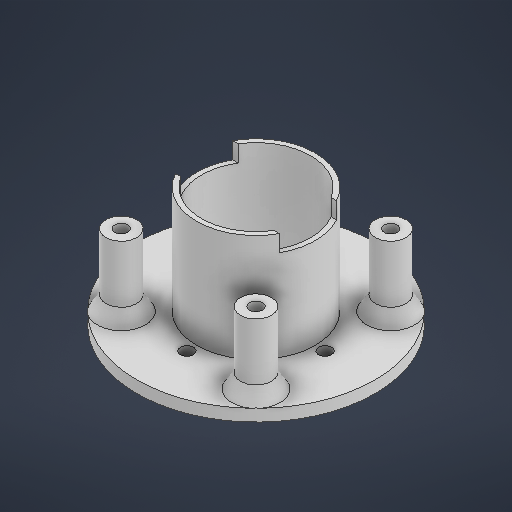
# Autodesk Inventor part: holder
Saved by Autodesk Inventor 2025 (Build 290162000, 162)
## iProperties
Created: 2024-10-04
Part Number: holder
Material: Generic
Document SubType Name: Modeling
Designer: mayhe
Density: 1 g/cm^3
Appearance: Default
Author: mayhe
Autodesk Inventor part; units mm, degrees
ref_plane "YZ Plane" through (0, 0, 0) normal (1, 0, 0) x (0, 1, 0)
ref_plane "XZ Plane" through (0, 0, 0) normal (0, 1, 0) x (-1, 0, 0)
ref_plane "XY Plane" through (0, 0, 0) normal (0, 0, 1) x (1, 0, 0)
sketch "Sketch1" plane through (0, 0, 0) normal (0, 1, 0) x (-1, 0, 0)
  circle A0 centre (0, 0) radius 50
  circle A1 centre (0, 0) radius 40
  circle A2 centre (0, -40) radius 2.75
  circle A3 centre (28.2843, -28.2843) radius 2.75
  circle A4 centre (40, 0) radius 2.75
  circle A5 centre (28.2843, 28.2843) radius 2.75
  circle A6 centre (0, 0) radius 22.9
  circle A7 centre (0, 0) radius 24.9
  line L0 (31.0901, 12) -> (-31.0901, 12)
  line L1 (-31.0901, 12) -> (-31.0901, -12)
  line L2 (-31.0901, -12) -> (31.0901, -12)
  line L3 (31.0901, -12) -> (31.0901, 12)
  line L4 (31.0901, 12) -> (-31.0901, -12) construction
  line L5 (-31.0901, 12) -> (31.0901, -12) construction
  circle A8 centre (0, 40) radius 2.75
  circle A9 centre (-28.2843, 28.2843) radius 2.75
  circle A10 centre (-40, 0) radius 2.75
  circle A11 centre (-28.2843, -28.2843) radius 2.75
  point P0 (-21.8177, 12)
  point P1 (-19.5041, 12)
  point P2 (19.5041, 12)
  point P3 (21.8177, 12)
  point P4 (21.8177, -12)
  point P5 (19.5041, -12)
  point P6 (-19.5041, -12)
  point P7 (-21.8177, -12)
  dimension "d1" = 80
  dimension "d0" = 100
  dimension "d2" = 5.5
  dimension "d5" = 360
  dimension "d7" = 45.8
  dimension "d8" = 2
  dimension "d9" = 24
  constraints: 12 end point, 11 centre point, 3 coincident, 2 midpoint, 2 parallel, 1 horizontal, 1 perpendicular, 1 vertical alignment, 19 other
  measures "d0" diameter of A0
  measures "d2" diameter of A2
  measures "d7" diameter of A6
  measures "d8" radial gap between concentric circles of A6 A7
  measures "d9" distance of L1.end L0.end
extrude "Extrusion1" add sketch "Sketch1" along normal blind 5 contours A0 | A1 A4 | A1 A4 | A4 A1 A3 A2 A11 A10 A9 A8 A5 | A8 A1 | A1 A8 | A2 A1 | A1 A2 | A10 A1 | A1 A10 | A6 L2 L0 | A6 L0 A7 L2 | L0 A6 | A6 L0 A7 | L2 A7 A6 | A6 L2 | A6 L2 A7 L0 | L0 L3 L2 A7 | A7 L2 L1 L0
extrude "Extrusion2" add sketch "Sketch1" along normal blind 50.1 contours A6 L0 A7 | L2 A7 A6
extrude "Extrusion3" add sketch "Sketch1" along normal blind 43.1 contours A6 L0 A7 L2 | A6 L2 A7 L0
sketch "Sketch2" plane through (0, 5, 0) normal (0, 1, 0) x (1, 0, 0)
  circle A0 centre (0, 0) radius 29
  circle A1 centre (29, 0) radius 2.75
  circle A2 centre (0, 29) radius 2.75
  circle A3 centre (-29, 0) radius 2.75
  circle A4 centre (0, -29) radius 2.75
  dimension "d16" = 58
  dimension "d17" = 5.5
  dimension "d20" = 360
  constraints: 4 centre point, 1 coincident, 1 horizontal alignment, 11 other
  measures "d17" diameter of A1
extrude "Extrusion4" cut sketch "Sketch2" against normal blind 43.1 contours A0 A1 | A0 A1 | A2 A0 | A0 A2 | A4 A0 | A0 A4 | A3 A0 | A0 A3
sketch "Sketch3" plane through (0, 5, 0) normal (0, 1, 0) x (1, 0, 0)
  circle A0 centre (-28.2843, 28.2843) radius 2.75 projected
  circle A1 centre (0, 0) radius 40
  circle A2 centre (0, 40) radius 6.5
  circle A3 centre (0, 40) radius 4
  line L0 (2.3094, 44) -> (4.6188, 40)
  line L1 (4.6188, 40) -> (2.3094, 36)
  line L2 (2.3094, 36) -> (-2.3094, 36)
  line L3 (-2.3094, 36) -> (-4.6188, 40)
  line L4 (-4.6188, 40) -> (-2.3094, 44)
  line L5 (-2.3094, 44) -> (2.3094, 44)
  circle A4 centre (-28.2843, 28.2843) radius 6.5
  line L6 (-29.4797, 32.7457) -> (-25.0183, 31.5503)
  line L7 (-32.7457, 29.4797) -> (-29.4797, 32.7457)
  line L8 (-31.5503, 25.0183) -> (-32.7457, 29.4797)
  circle A5 centre (-28.2843, 28.2843) radius 4
  line L9 (-25.0183, 31.5503) -> (-23.8229, 27.0888)
  line L10 (-23.8229, 27.0888) -> (-27.0888, 23.8229)
  line L11 (-27.0888, 23.8229) -> (-31.5503, 25.0183)
  circle A6 centre (-40, 0) radius 6.5
  line L12 (-44, 2.3094) -> (-40, 4.6188)
  line L13 (-44, -2.3094) -> (-44, 2.3094)
  line L14 (-40, -4.6188) -> (-44, -2.3094)
  circle A7 centre (-40, 0) radius 4
  line L15 (-40, 4.6188) -> (-36, 2.3094)
  line L16 (-36, 2.3094) -> (-36, -2.3094)
  line L17 (-36, -2.3094) -> (-40, -4.6188)
  circle A8 centre (-28.2843, -28.2843) radius 6.5
  line L18 (-32.7457, -29.4797) -> (-31.5503, -25.0183)
  line L19 (-29.4797, -32.7457) -> (-32.7457, -29.4797)
  line L20 (-25.0183, -31.5503) -> (-29.4797, -32.7457)
  circle A9 centre (-28.2843, -28.2843) radius 4
  line L21 (-31.5503, -25.0183) -> (-27.0888, -23.8229)
  line L22 (-27.0888, -23.8229) -> (-23.8229, -27.0888)
  line L23 (-23.8229, -27.0888) -> (-25.0183, -31.5503)
  circle A10 centre (0, -40) radius 6.5
  line L24 (-2.3094, -44) -> (-4.6188, -40)
  line L25 (2.3094, -44) -> (-2.3094, -44)
  line L26 (4.6188, -40) -> (2.3094, -44)
  circle A11 centre (0, -40) radius 4
  line L27 (-4.6188, -40) -> (-2.3094, -36)
  line L28 (-2.3094, -36) -> (2.3094, -36)
  line L29 (2.3094, -36) -> (4.6188, -40)
  circle A12 centre (28.2843, -28.2843) radius 6.5
  line L30 (29.4797, -32.7457) -> (25.0183, -31.5503)
  line L31 (32.7457, -29.4797) -> (29.4797, -32.7457)
  line L32 (31.5503, -25.0183) -> (32.7457, -29.4797)
  circle A13 centre (28.2843, -28.2843) radius 4
  line L33 (25.0183, -31.5503) -> (23.8229, -27.0888)
  line L34 (23.8229, -27.0888) -> (27.0888, -23.8229)
  line L35 (27.0888, -23.8229) -> (31.5503, -25.0183)
  circle A14 centre (40, 0) radius 6.5
  line L36 (44, -2.3094) -> (40, -4.6188)
  line L37 (44, 2.3094) -> (44, -2.3094)
  line L38 (40, 4.6188) -> (44, 2.3094)
  circle A15 centre (40, 0) radius 4
  line L39 (40, -4.6188) -> (36, -2.3094)
  line L40 (36, -2.3094) -> (36, 2.3094)
  line L41 (36, 2.3094) -> (40, 4.6188)
  circle A16 centre (28.2843, 28.2843) radius 6.5
  line L42 (32.7457, 29.4797) -> (31.5503, 25.0183)
  line L43 (29.4797, 32.7457) -> (32.7457, 29.4797)
  line L44 (25.0183, 31.5503) -> (29.4797, 32.7457)
  circle A17 centre (28.2843, 28.2843) radius 4
  line L45 (31.5503, 25.0183) -> (27.0888, 23.8229)
  line L46 (27.0888, 23.8229) -> (23.8229, 27.0888)
  line L47 (23.8229, 27.0888) -> (25.0183, 31.5503)
  circle A18 centre (40, 0) radius 2.75
  circle A19 centre (28.2843, 28.2843) radius 2.75
  circle A20 centre (0, 40) radius 2.75
  circle A21 centre (-28.2843, 28.2843) radius 2.75
  circle A22 centre (-40, 0) radius 2.75
  circle A23 centre (-28.2843, -28.2843) radius 2.75
  circle A24 centre (0, -40) radius 2.75
  circle A25 centre (28.2843, -28.2843) radius 2.75
  point P0 (0, 44)
  point P1 (-31.1127, 31.1127)
  point P2 (-44, 0)
  point P3 (-31.1127, -31.1127)
  point P4 (0, -44)
  point P5 (31.1127, -31.1127)
  point P6 (44, 0)
  point P7 (31.1127, 31.1127)
  point P8 (-4.4739, 39.749)
  point P9 (-3.4641, 38)
  point P10 (-3.995, 39.8)
  dimension "d29" = 8
  dimension "d24" = 13
  dimension "d36" = 360
  dimension "d38" = 5.5
  dimension "d41" = 360
  constraints: 96 end point, 17 centre point, 11 coincident, 2 horizontal alignment, 2 point on circle, 1 midpoint, 1 vertical alignment, 188 other
  measures "d24" diameter of A2
  measures "d38" diameter of A18
extrude "Extrusion5" add sketch "Sketch3" along normal blind 15 contours A0 A1 A5 | A0 A1 A5 | A5 L6 L9 A1 | A1 L9 A5 | A5 L11 A1 | A1 L11 L8 A5 | L9 L6 L7 L8 L11 A1 A4 | A1 A4 L11 L10 L9 | L9 L10 A5 | A5 L7 L6 | L8 L7 A5 | A5 L10 L11 | A16 A1 L45 L42 L43 L44 L47 | A1 L47 L46 L45 A16 | A8 A1 L23 L22 L21 | A1 L21 L18 L19 L20 L23 A8 | L47 L44 A17 A1 | A1 A17 L47 | L21 A9 A1 | A1 A9 L18 L21 | A17 A1 A19 | A1 A19 A17 | A17 L46 L47 | L45 A17 A1 | A1 A17 L42 L45 | A9 A1 A23 | A1 A23 A9 | L21 L22 A9 | L23 L20 A9 A1 | A1 A9 L23 | L44 L43 A17 | A17 L45 L46 | A9 L19 L18 | L22 L23 A9 | L43 L42 A17 | A12 A1 L33 L30 L31 L32 L35 | A1 L35 L34 L33 A12 | A9 L20 L19 | L35 L32 A13 A1 | A1 A13 L35 | L33 A13 A1 | A1 A13 L30 L33 | A13 A1 A25 | A1 A25 A13 | A13 L34 L35 | L33 L34 A13 | L32 L31 A13 | A13 L31 L30
sketch "Sketch4" plane through (28.2843, 20, 28.2843) normal (0, 1, 0) x (1, 0, 0)
  circle A0 centre (0, 0) radius 6.5 projected
  circle A1 centre (0, 0) radius 6.5
  circle A2 centre (0, 0) radius 4
  circle A3 centre (0, 0) radius 2.75
  line L0 (4, -2.3094) -> (0, -4.6188)
  line L1 (0, -4.6188) -> (-4, -2.3094)
  line L2 (-4, -2.3094) -> (-4, 2.3094)
  line L3 (-4, 2.3094) -> (0, 4.6188)
  line L4 (0, 4.6188) -> (4, 2.3094)
  line L5 (4, 2.3094) -> (4, -2.3094)
  circle A4 centre (-28.2843, 28.2843) radius 40
  circle A5 centre (11.7157, 28.2843) radius 6.5
  line L6 (8.4497, 31.5503) -> (12.9112, 32.7457)
  line L7 (7.2543, 27.0888) -> (8.4497, 31.5503)
  line L8 (10.5203, 23.8229) -> (7.2543, 27.0888)
  line L9 (14.9817, 25.0183) -> (10.5203, 23.8229)
  line L10 (16.1771, 29.4797) -> (14.9817, 25.0183)
  line L11 (12.9112, 32.7457) -> (16.1771, 29.4797)
  circle A6 centre (11.7157, 28.2843) radius 2.75
  circle A7 centre (0, 56.5685) radius 6.5
  line L12 (-4.6188, 56.5685) -> (-2.3094, 60.5685)
  line L13 (-2.3094, 52.5685) -> (-4.6188, 56.5685)
  line L14 (2.3094, 52.5685) -> (-2.3094, 52.5685)
  line L15 (4.6188, 56.5685) -> (2.3094, 52.5685)
  line L16 (2.3094, 60.5685) -> (4.6188, 56.5685)
  line L17 (-2.3094, 60.5685) -> (2.3094, 60.5685)
  circle A8 centre (0, 56.5685) radius 2.75
  circle A9 centre (-28.2843, 68.2843) radius 6.5
  line L18 (-31.5503, 65.0183) -> (-32.7457, 69.4797)
  line L19 (-27.0888, 63.8229) -> (-31.5503, 65.0183)
  line L20 (-23.8229, 67.0888) -> (-27.0888, 63.8229)
  line L21 (-25.0183, 71.5503) -> (-23.8229, 67.0888)
  line L22 (-29.4797, 72.7457) -> (-25.0183, 71.5503)
  line L23 (-32.7457, 69.4797) -> (-29.4797, 72.7457)
  circle A10 centre (-28.2843, 68.2843) radius 2.75
  circle A11 centre (-56.5685, 56.5685) radius 6.5
  line L24 (-56.5685, 51.9497) -> (-60.5685, 54.2591)
  line L25 (-52.5685, 54.2591) -> (-56.5685, 51.9497)
  line L26 (-52.5685, 58.8779) -> (-52.5685, 54.2591)
  line L27 (-56.5685, 61.1873) -> (-52.5685, 58.8779)
  line L28 (-60.5685, 58.8779) -> (-56.5685, 61.1873)
  line L29 (-60.5685, 54.2591) -> (-60.5685, 58.8779)
  circle A12 centre (-56.5685, 56.5685) radius 2.75
  circle A13 centre (-68.2843, 28.2843) radius 6.5
  line L30 (-65.0183, 25.0183) -> (-69.4797, 23.8229)
  line L31 (-63.8229, 29.4797) -> (-65.0183, 25.0183)
  line L32 (-67.0888, 32.7457) -> (-63.8229, 29.4797)
  line L33 (-71.5503, 31.5503) -> (-67.0888, 32.7457)
  line L34 (-72.7457, 27.0888) -> (-71.5503, 31.5503)
  line L35 (-69.4797, 23.8229) -> (-72.7457, 27.0888)
  circle A14 centre (-68.2843, 28.2843) radius 2.75
  circle A15 centre (-56.5685, 0) radius 6.5
  line L36 (-51.9497, 0) -> (-54.2591, -4)
  line L37 (-54.2591, 4) -> (-51.9497, 0)
  line L38 (-58.8779, 4) -> (-54.2591, 4)
  line L39 (-61.1873, 0) -> (-58.8779, 4)
  line L40 (-58.8779, -4) -> (-61.1873, 0)
  line L41 (-54.2591, -4) -> (-58.8779, -4)
  circle A16 centre (-56.5685, 0) radius 2.75
  circle A17 centre (-28.2843, -11.7157) radius 6.5
  line L42 (-25.0183, -8.4497) -> (-23.8229, -12.9112)
  line L43 (-29.4797, -7.2543) -> (-25.0183, -8.4497)
  line L44 (-32.7457, -10.5203) -> (-29.4797, -7.2543)
  line L45 (-31.5503, -14.9817) -> (-32.7457, -10.5203)
  line L46 (-27.0888, -16.1771) -> (-31.5503, -14.9817)
  line L47 (-23.8229, -12.9112) -> (-27.0888, -16.1771)
  circle A18 centre (-28.2843, -11.7157) radius 2.75
  point P0 (4, 0)
  point P1 (14.5442, 31.1127)
  point P2 (0, 60.5685)
  point P3 (-31.1127, 71.1127)
  point P4 (-60.5685, 56.5685)
  point P5 (-71.1127, 25.4558)
  point P6 (-56.5685, -4)
  point P7 (-25.4558, -14.5442)
  dimension "d45" = 8
  dimension "d48" = 360
  constraints: 96 end point, 16 centre point, 5 coincident, 1 horizontal alignment, 1 midpoint, 155 other
extrude "Extrusion6" add sketch "Sketch4" along normal blind 5 contours A0 A4 L1 L0 L5 L4 | A4 L4 L3 L2 L1 A0 | A7 A4 L12 L13 L14 L15 | A4 L15 L16 L17 L12 A7 | A15 A4 L39 L40 L41 L36 | A4 L36 L37 L38 L39 A15 | A11 A4 L24 L25 L26 L27 | A4 L27 L28 L29 L24 A11
sketch "Sketch5" plane through (28.2843, 25, 28.2843) normal (0, 1, 0) x (1, 0, 0)
  circle A0 centre (0, 0) radius 2.75 projected
  circle A1 centre (-28.2843, 28.2843) radius 40
  circle A2 centre (-56.5685, 0) radius 2.75 projected
  circle A3 centre (-56.5685, 0) radius 6.5
  circle A4 centre (-56.5685, 56.5685) radius 6.5 projected
  circle A5 centre (-56.5685, 56.5685) radius 6.5
  circle A6 centre (0, 56.5685) radius 6.5 projected
  circle A7 centre (0, 56.5685) radius 6.5
  circle A8 centre (0, 0) radius 6.5 projected
  circle A9 centre (0, 0) radius 6.5
  circle A10 centre (0, 0) radius 2.75
  circle A11 centre (11.7157, 28.2843) radius 6.5
  circle A12 centre (11.7157, 28.2843) radius 2.75
  circle A13 centre (0, 56.5685) radius 6.5
  circle A14 centre (0, 56.5685) radius 2.75
  circle A15 centre (-28.2843, 68.2843) radius 6.5
  circle A16 centre (-28.2843, 68.2843) radius 2.75
  circle A17 centre (-56.5685, 56.5685) radius 6.5
  circle A18 centre (-56.5685, 56.5685) radius 2.75
  circle A19 centre (-68.2843, 28.2843) radius 6.5
  circle A20 centre (-68.2843, 28.2843) radius 2.75
  circle A21 centre (-56.5685, 0) radius 6.5
  circle A22 centre (-56.5685, 0) radius 2.75
  circle A23 centre (-28.2843, -11.7157) radius 6.5
  circle A24 centre (-28.2843, -11.7157) radius 2.75
  dimension "d52" = 5.5
  dimension "d55" = 360
  constraints: 19 centre point, 13 coincident, 36 other
  measures "d52" diameter of A10
extrude "Extrusion7" add sketch "Sketch5" along normal blind 10 contours A0 A1 A8 | A0 A1 A8 | A6 A1 A14 | A1 A14 A6 | A3 A1 A2 | A1 A2 A3 | A4 A1 A18 | A1 A18 A4
chamfer "Chamfer1" distance 3.5875 distance2 6 4 edges at (21.7843, 5, 28.2843) (21.7843, 5, -28.2843) (-34.7843, 5, -28.2843) (-34.7843, 5, 28.2843)
body "Solid1"
